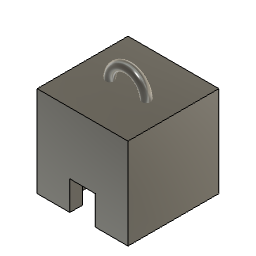
2023_09_29_Kyb_Kalman_Eggdrop v2 (Autodesk Fusion 360 design; units mm, degrees)
Autodesk Fusion 360 part; units mm, degrees
sketch "Sketch1" plane through (0, 0, 0) normal (0, 0, 1) x (1, 0, 0)
  line L0 (0, 0) -> (50, 0)
  line L1 (50, 0) -> (50, 50)
  line L2 (50, 50) -> (0, 50)
  line L3 (0, 50) -> (0, 0)
  constraint horizontal L0
  constraint vertical L1
  constraint horizontal L2
  constraint vertical L3
  constraint coincident L0.start L3.end
extrude "Extrude1" add sketch "Sketch1" along normal blind 40 makes body 1
extrude "Extrude2" add 1 faces at (16.6667, 33.3333, 40) along direction (0, 0, 1) blind 10 on bodies 1 bodies 1
sketch "Sketch2" plane through (0, 0, 0) normal (0, 0, -1) x (1, 0, 0)
  line L0 (0, 0) -> (0, -50)
  line L1 (0, -50) -> (50, -50)
  line L2 (50, -50) -> (50, 0)
  line L3 (50, 0) -> (0, 0)
  line L4 (39, -43) -> (11, -43)
  line L5 (11, -43) -> (11, -7)
  line L6 (11, -7) -> (39, -7)
  line L7 (39, -7) -> (39, -43)
  line L8 (32, -7) -> (18, -7)
  line L9 (18, -7) -> (18, 0)
  line L10 (18, 0) -> (32, 0)
  line L11 (32, 0) -> (32, -7)
  circle A0 centre (35, -19) radius 2.5
  circle A1 centre (15, -19) radius 2.5
  dimension "d5" = 5
  dimension "d6" = 5
  constraint horizontal L4
  constraint vertical L5
  constraint horizontal L6
  constraint vertical L7
  constraint horizontal L8
  constraint vertical L9
  constraint horizontal L10
  constraint vertical L11
  constraint coincident L3 L9.end
  constraint coincident L6 L8.start
  measures "d5" diameter of A0
  measures "d6" diameter of A1
extrude "Extrude3" cut sketch "Sketch2" against normal blind 16 contours L3 L6 L8 L9 L10 L11 | L4 L5 L6 L7 L8 | A0 | A1 bodies 1
torus "TorusPrimitive1" add centre line diameter 20 section diameter 7 placed x (1, 0, 0) y (0, 0, 1) z (0, -1, 0) at (25, 0, 50) bodies 1
move_face "MoveFace1" to x (1, 0, 0) y (0, 1, 0) z (0, 0, 1) at (0, 31, 0) 1 faces at (11.5861, 0.6935, 50.6695) on bodies 1
move_face "MoveFace2" to x (1, 0, 0) y (0, 1, 0) z (0, 0, 1) at (0, 3, 0) 1 faces at (11.5861, 0.6935, 50.6695) on bodies 1
move_face "MoveFace3" to x (1, 0, 0) y (0, 1, 0) z (0, 0, 1) at (0, 3, 0) 1 faces at (11.5861, 3.6935, 50.6695) on bodies 1
delete_face "DeleteFace1" 1 faces at (11.5861, 3.6935, 50.6695) on bodies 1
torus "TorusPrimitive2" add centre line diameter 30 section diameter 7 placed x (1, 0, 0) y (0, 0, 1) z (0, -1, 0) at (25, 0, 50) bodies 1
move_face "MoveFace4" to x (1, 0, 0) y (0, 1, 0) z (0, 0, 1) at (0, -6, 0) 1 faces at (6.5639, -0.6607, 49.8118) on bodies 1
delete_face "DeleteFace2" 1 faces at (6.5639, -0.6607, 49.8118) on bodies 1
torus "TorusPrimitive3" add centre line diameter 20 section diameter 5 placed x (1, 0, 0) y (0, 0, -1) z (0, 1, 0) at (10, 0, 10) separate body makes body 2
move_body "MoveFace5" bodies 2 to x (1, 0, 0) y (0, 1, 0) z (0, 0, 1) at (15, 25, 40) on bodies 2
extrude "Extrude4" add sketch "Sketch2" against normal blind 16 contours A0 | A1 bodies 1
extrude "Extrude5" cut sketch "Sketch2" against normal blind 21 contours A0 | A1 bodies 1
thread "Thread1" "ISO Metric profile 4.0 M4x0.7 6H" major diameter 4.1095 minor diameter 3.332 pitch 0.7 angle 60 resizes the face on face at (17.4876, 19.2489, 17.6667) on bodies 1
thread "Thread2" "ISO Metric profile 5.0 M5x0.8 6H" major diameter 5.12 minor diameter 4.234 pitch 0.8 angle 60 resizes the face on face at (37.4876, 19.2489, 17.6667) on bodies 1
extrude "Extrude6" cut 2 faces at (34.7422, 18.3431, 21) (15.4892, 19.3901, 21) along direction (0, 0, 1) blind 5 on bodies 1 bodies 1
thread "Thread3" "ISO Metric profile 4.0 M4x0.7 6H" major diameter 4.1095 minor diameter 3.332 pitch 0.7 angle 60 resizes the face on face at (34.6324, 16.9152, 19.3333) on face at (34.6324, 16.9152, 22.6667) on bodies 1
